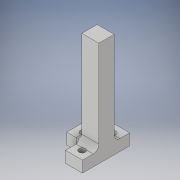
# Autodesk Inventor part: SolarpanelHalterung
Saved by Autodesk Inventor 2018 (Build 220112000, 112)
## iProperties
Created: 2018-04-27
Part Number: SolarpanelHalterung
Material: Generisch
Document SubType Name: Modeling
Designer: gchri
Density: 1 g/cm^3
Appearance: Vorgabe
Author: gchri
Autodesk Inventor part; units mm, degrees
ref_plane "YZ Plane" through (0, 0, 0) normal (1, 0, 0) x (0, 1, 0)
ref_plane "XZ Plane" through (0, 0, 0) normal (0, 1, 0) x (-1, 0, 0)
ref_plane "XY Plane" through (0, 0, 0) normal (0, 0, 1) x (1, 0, 0)
sketch "Skizze1" plane through (0, 0, 0) normal (0, 0, 1) x (1, 0, 0)
  line L0 (-116.7202, -92.2798) -> (-131.7202, -107.2798) projected
  line L1 (-131.7202, -107.2798) -> (-131.7202, -92.2798) projected
  line L2 (-131.7202, -92.2798) -> (-116.7202, -92.2798) projected
  circle A0 centre (-156.7202, -88.2798) radius 1.7 projected
  circle A1 centre (-136.7202, -152.4798) radius 1.7 projected
  circle A2 centre (-156.7202, -152.4798) radius 1.7 projected
  circle A3 centre (-156.7202, -126.4798) radius 1.7 projected
  circle A4 centre (-136.7202, -126.4798) radius 1.7 projected
  circle A5 centre (-138.7202, -101.5941) radius 1.7 projected
  circle A6 centre (-154.7202, -101.5941) radius 1.7 projected
  circle A7 centre (-146.7202, -109.0302) radius 1.7 projected
  circle A8 centre (-92.4455, -87.0864) radius 1.7 projected
  line L3 (-116.7202, -2.2798) -> (-131.7202, 12.7202) projected
  line L4 (-131.7202, -2.2798) -> (-116.7202, -2.2798) projected
  line L5 (-131.7202, 12.7202) -> (-131.7202, -2.2798) projected
  circle A9 centre (-156.7202, -6.2798) radius 1.7 projected
  circle A10 centre (-136.7202, 57.9202) radius 1.7 projected
  circle A11 centre (-156.7202, 57.9202) radius 1.7 projected
  circle A12 centre (-156.7202, 31.9202) radius 1.7 projected
  circle A13 centre (-136.7202, 31.9202) radius 1.7 projected
  circle A14 centre (-138.7202, 7.0345) radius 1.7 projected
  circle A15 centre (-154.7202, 7.0345) radius 1.7 projected
  circle A16 centre (-146.7202, 14.4706) radius 1.7 projected
  circle A17 centre (-92.4455, -7.4732) radius 1.7 projected
  line L6 (-6.7202, -92.2798) -> (8.2798, -107.2798) projected
  line L7 (8.2798, -92.2798) -> (-6.7202, -92.2798) projected
  line L8 (8.2798, -107.2798) -> (8.2798, -92.2798) projected
  circle A18 centre (33.2798, -88.2798) radius 1.7 projected
  circle A19 centre (13.2798, -152.4798) radius 1.7 projected
  circle A20 centre (33.2798, -152.4798) radius 1.7 projected
  circle A21 centre (33.2798, -126.4798) radius 1.7 projected
  circle A22 centre (13.2798, -126.4798) radius 1.7 projected
  circle A23 centre (15.2798, -101.5941) radius 1.7 projected
  circle A24 centre (31.2798, -101.5941) radius 1.7 projected
  circle A25 centre (23.2798, -109.0302) radius 1.7 projected
  circle A26 centre (-30.9949, -87.0864) radius 1.7 projected
  line L9 (-16.7202, -2.2798) -> (-106.7202, -2.2798) projected
  line L10 (-131.7202, 22.7202) -> (-106.7202, -2.2798) projected
  line L11 (-131.7202, 70.2202) -> (-131.7202, 22.7202) projected
  line L12 (-131.7202, 70.2202) -> (-161.7202, 70.2202) projected
  line L13 (-161.7202, -164.7798) -> (-161.7202, 70.2202) projected
  line L14 (-131.7202, -164.7798) -> (-161.7202, -164.7798) projected
  line L15 (-131.7202, -164.7798) -> (-131.7202, -117.2798) projected
  line L16 (-131.7202, -117.2798) -> (-106.7202, -92.2798) projected
  line L17 (-106.7202, -92.2798) -> (-16.7202, -92.2798) projected
  line L18 (8.2798, -117.2798) -> (-16.7202, -92.2798) projected
  line L19 (8.2798, -164.7798) -> (8.2798, -117.2798) projected
  line L20 (8.2798, -164.7798) -> (38.2798, -164.7798) projected
  line L21 (38.2798, 70.2202) -> (38.2798, -164.7798) projected
  line L22 (8.2798, 70.2202) -> (38.2798, 70.2202) projected
  line L23 (8.2798, 70.2202) -> (8.2798, 22.7202) projected
  line L24 (8.2798, 22.7202) -> (-16.7202, -2.2798) projected
  circle A27 centre (-30.9949, -7.4732) radius 1.7 projected
  circle A28 centre (23.2798, 14.4706) radius 1.7 projected
  circle A29 centre (31.2798, 7.0345) radius 1.7 projected
  circle A30 centre (15.2798, 7.0345) radius 1.7 projected
  circle A31 centre (13.2798, 31.9202) radius 1.7 projected
  circle A32 centre (33.2798, 31.9202) radius 1.7 projected
  circle A33 centre (33.2798, 57.9202) radius 1.7 projected
  circle A34 centre (13.2798, 57.9202) radius 1.7 projected
  circle A35 centre (33.2798, -6.2798) radius 1.7 projected
  line L25 (-6.7202, -2.2798) -> (8.2798, 12.7202) projected
  line L26 (8.2798, 12.7202) -> (8.2798, -2.2798) projected
  line L27 (8.2798, -2.2798) -> (-6.7202, -2.2798) projected
  line L28 (18.7798, 18.9706) -> (27.7798, 18.9706)
  line L29 (27.7798, -6.0294) -> (18.7798, -6.0294)
  line L30 (35.7798, 10.772) -> (35.7798, 2.6465)
  line L31 (10.7798, 2.6465) -> (10.7798, 10.772)
  line L32 (18.7798, -6.0294) -> (18.7798, 2.6465)
  line L33 (18.7798, 10.772) -> (18.7798, 18.9706)
  line L34 (10.7798, 10.772) -> (18.7798, 10.772)
  line L35 (27.7798, 10.772) -> (35.7798, 10.772)
  line L36 (27.7798, 18.9706) -> (27.7798, 10.772)
  line L37 (27.7798, 2.6465) -> (27.7798, -6.0294)
  line L38 (35.7798, 2.6465) -> (27.7798, 2.6465)
  line L39 (18.7798, 2.6465) -> (10.7798, 2.6465)
  circle A36 centre (23.2798, -1.6915) radius 1.7
  point P0 (0, 0)
  dimension "d0" = 9
  dimension "d1" = 25
  dimension "d2" = 4.5
  dimension "d4" = 25
  dimension "d21" = 3.4
  constraints: 24 end point, 10 parallel, 4 perpendicular, 3 horizontal, 1 centre point
  measures "d0" distance of L29.start L29.end
  measures "d1" distance of L28.end L29.start
  measures "d2" distance from line of L28 A28.centre
  measures "d4" distance of L30.end L31.start
  measures "d21" diameter of A36
extrude "Extrusion1" add sketch "Skizze1" along normal blind 75 contours L28 L36 L35 L30 L38 L37 L29 L32 L39 L31 L34 L33
sketch "Skizze2" plane through (18.7798, 10.772, 0) normal (-1, 0, 0) x (0, 0, 1)
  line L0 (0, 0) -> (0, 8.1985) projected
  line L1 (0, 0) -> (75, 0) projected
  line L2 (75, 8.1985) -> (75, 0) projected
  line L3 (0, 8.1985) -> (75, 8.1985) projected
  line L4 (0, -16.8015) -> (0, -8.1255) projected
  line L5 (0, -16.8015) -> (75, -16.8015) projected
  line L6 (75, -8.1255) -> (75, -16.8015) projected
  line L7 (0, -8.1255) -> (75, -8.1255) projected
  line L8 (0, 8.1985) -> (75, 8.1985) projected
  line L9 (6, 8.1985) -> (6, 0)
  line L10 (6, -8.1255) -> (6, -16.8015)
  point P0 (0, -10.772)
  dimension "d8" = 6
  constraints: 4 end point, 4 point on line, 1 perpendicular, 1 vertical
  measures "d8" distance between parallel lines of L0 L9
extrude "Extrusion2" cut sketch "Skizze2" against normal blind 75 contours L9 L3 L2 L1 | L10 L7 L6 L5
sketch "Skizze3" plane through (27.7798, 10.772, 0) normal (0, 1, 0) x (1, 0, 0)
  line L0 (-9, 0) -> (-9, -6) projected
  line L1 (-9, -6) -> (-17.0308, -6)
  line L2 (8, 0) -> (8, -75) projected
  line L3 (0, 0) -> (8, 0) projected
  line L4 (0, 0) -> (0, -6) projected
  line L5 (-9, -6) -> (0, -6) projected
  line L6 (-9, 0) -> (-9, -6) projected
  line L7 (-17, 0) -> (-9, 0) projected
  line L8 (-17, 0) -> (-17, -75) projected
  line L9 (8, -75) -> (-17, -75) projected
  line L10 (0, -6) -> (8, -6)
  line L11 (8, 0) -> (8, -75) projected
  arc A0 (-17, -5.991) -> (-17.0308, -6) centre (-15.2533, -11.9955) ccw
  circle A1 centre (-3.7054, -68.1948) radius 6 projected
  circle A2 centre (-3.7054, -68.1948) radius 3 projected
  line L12 (-17, 0) -> (-17, -75) projected
  line L13 (-17, 0) -> (-17, -75) projected
  line L14 (-17, -59.7256) -> (8, -59.7256)
  line L15 (-9, -6) -> (-9, -59.7256)
  line L16 (0, -6) -> (0, -59.7256)
  line L17 (-17, -5.991) -> (-9, -5.991)
  line L18 (-9, -5.991) -> (-9, -59.7256)
  line L19 (-9, -59.7256) -> (-17, -59.7256)
  line L20 (-17, -59.7256) -> (-17, -5.991)
  line L21 (0, -59.7256) -> (8, -59.7256)
  line L22 (8, -59.7256) -> (8, -6)
  line L23 (8, -6) -> (0, -6)
  line L24 (0, -6) -> (0, -59.7256)
  line L25 (-17, -59.7256) -> (-17, -75)
  line L26 (-17, -75) -> (8, -75)
  line L27 (8, -59.7256) -> (8, -75)
  arc A3 (-17, -62.5279) -> (-5.3377, -75) centre (-4.4998, -62.5279) ccw
  arc A4 (-3.6671, -75) -> (8, -62.5279) centre (-4.4998, -62.5279) ccw
  circle A5 centre (-4.4998, -68.1948) radius 2.6
  point P0 (-27.7798, 0)
  dimension "d14" = 5.2
  constraints: 32 end point, 10 point on line, 7 perpendicular, 6 point on circle, 4 centre point, 4 parallel, 3 horizontal, 2 collinear, 2 tangent
  measures "d14" diameter of A5
extrude "Extrusion3" cut sketch "Skizze3" against normal blind 75 contours L0 L1 L8 L17 | L15 L14 L8 L1 | L10 L2 L14 L16 | A3 L9 L8 | L2 L9 A4 | A5 A2 | A2 A5 picked at (-5.1031, -67.7544) picked at (-6.7866, -68.6249)
fillet "Rundung2" radius 3 8 edges at (27.7798, 6.7093, 6) (23.2798, 10.772, 6) (18.7798, 6.7093, 5.991) (23.2798, 2.6465, 6) (27.7798, 2.6465, 3) (27.7798, 10.772, 3) (18.7798, 10.772, 2.9955) (18.7798, 2.6465, 2.9955)
sketch "Skizze4" plane through (22.4421, 2.6465, 75) normal (0, -1, 0) x (1, 0, 0)
  line L0 (-17.772, 3.6645) -> (19.2771, 3.6645)
  line L1 (19.2771, 3.6645) -> (19.2771, -19.6858)
  line L2 (19.2771, -19.6858) -> (-17.772, -19.6858)
  line L3 (-17.772, -19.6858) -> (-17.772, 3.6645)
  point P0 (-22.4421, -75)
  constraints: 8 end point, 2 parallel, 1 horizontal, 1 perpendicular
extrude "Extrusion4" cut sketch "Skizze4" against normal blind 10
sketch "Skizze5" plane through (18.7798, -6.0294, 0) normal (0, -1, 0) x (1, 0, 0)
  line L0 (9, 9) -> (9, 55.3142) projected
  line L1 (9, 14.3497) -> (19.6208, 14.3497)
  line L2 (19.6208, 14.3497) -> (19.6208, -3.739)
  line L3 (19.6208, -3.739) -> (9, -3.739)
  line L4 (9, -3.739) -> (9, 14.3497)
  point P0 (-18.7798, 0)
  constraints: 8 end point, 2 parallel, 1 horizontal, 1 perpendicular, 1 point on line
extrude "Extrusion5" cut sketch "Skizze5" against normal through all
